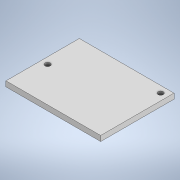
# Autodesk Inventor part: maestro_Subs
Saved by Autodesk Inventor 2020.1 (Build 241239000, 239)
## iProperties
Created: 2022-10-15
Part Number: maestro_Subs
Material: Generic
Document SubType Name: Modeling
Designer: OEM
Density: 1 g/cm^3
Appearance: Default
Author: OEM
Autodesk Inventor part; units mm, degrees
ref_plane "YZ Plane" through (0, 0, 0) normal (1, 0, 0) x (0, 1, 0)
ref_plane "XZ Plane" through (0, 0, 0) normal (0, 1, 0) x (-1, 0, 0)
ref_plane "XY Plane" through (0, 0, 0) normal (0, 0, 1) x (1, 0, 0)
sketch "Sketch1" plane through (0, 0, 0) normal (0, 1, 0) x (-1, 0, 0)
  line L0 (18.034, 13.97) -> (-18.034, 13.97)
  line L1 (-18.034, 13.97) -> (-18.034, -13.97)
  line L2 (-18.034, -13.97) -> (18.034, -13.97)
  line L3 (18.034, -13.97) -> (18.034, 13.97)
  line L4 (18.034, 13.97) -> (-18.034, -13.97) construction
  line L5 (-18.034, 13.97) -> (18.034, -13.97) construction
  circle A0 centre (-15.494, -11.43) radius 1
  circle A1 centre (15.494, 0.635) radius 1
  point P0 (0, 0)
  dimension "d0" = 27.94
  dimension "d1" = 36.068
  dimension "d3" = 2.54
  dimension "d4" = 2.54
  dimension "d5" = 13.335
  dimension "d6" = 2.54
  dimension "d7" = 2
  dimension "d8" = 2
  dimension "d11" = 30.988
  dimension "d12" = 12.065
  constraints: 12 end point, 2 centre point, 2 midpoint, 2 parallel, 1 horizontal, 1 perpendicular
  measures "d0" distance of L2.end L0.start
  measures "d1" distance of L1.end L2.end
  measures "d3" distance from line of L1 A0.centre
  measures "d4" distance from line of L2 A0.centre
  measures "d5" distance from line of L0 A1.centre
  measures "d6" distance from line of L3 A1.centre
  measures "d7" diameter of A1
  measures "d8" diameter of A0
  measures "d11" horizontal distance of A0.centre A1.centre
  measures "d12" vertical distance of A1.centre A0.centre
extrude "Extrusion1" add sketch "Sketch1" along normal blind 2
equation "\"d7\" = d8"
body "Solid1"
